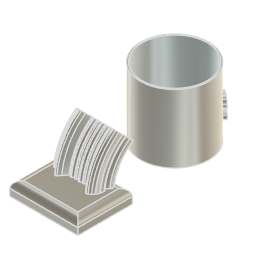
DecorativePieces (Autodesk Fusion 360 design; units mm, degrees)
Autodesk Fusion 360 part; units mm, degrees
(part 1 of 2)
sketch "Sketch1" plane through (0, 0, 0) normal (0, 0, 1) x (1, 0, 0)
  line L0 (50, 40) -> (-50, 40)
  line L1 (-50, 40) -> (-50, -40)
  line L2 (-50, -40) -> (50, -40)
  line L3 (50, -40) -> (50, 40)
  line L4 (50, 40) -> (-50, -40) construction
  line L5 (-50, 40) -> (50, -40) construction
  dimension "d1" = 100
  dimension "d2" = 80
  constraint horizontal L0
  constraint perpendicular L0 L1
  constraint parallel L0 L2
  constraint parallel L1 L3
  constraint coincident L4 origin
  constraint coincident L5 origin
  measures "d1" distance of L0.start L0.end
  measures "d2" distance of L0.end L1.end
extrude "Extrude1" add sketch "Sketch1" along normal blind 20 makes body 1
ref_plane "WorkPlane1" through (0, -40, 20) normal (0, 0.707107, 0.707107) x (1, 0, 0)
ref_plane "WorkPlane2" through (0, 30.7107, 90.7107) normal (0, 0.707107, 0.707107) x (1, 0, 0)
sketch "Sketch2" plane through (0, 60.7107, 60.7107) normal (0, 0.707107, 0.707107) x (1, 0, 0)
  line L0 (22.4639, -18.7054) -> (26.5034, -16.4275)
  spline S0 degree 2 poles (26.5034, -16.4275) (27.8398, -14.1648) (29.1838, -12.1526) knots 0 0 0 1 1 1
  spline S1 degree 2 poles (29.1838, -12.1526) (30.5277, -10.1405) (31.568, -8.8269) knots 0 0 0 1 1 1
  spline S2 degree 2 poles (31.568, -8.8269) (32.6082, -7.5133) (33.3675, -6.8223) knots 0 0 0 1 1 1
  spline S3 degree 2 poles (33.3675, -6.8223) (34.1268, -6.1314) (34.4913, -6.1314) knots 0 0 0 1 1 1
  spline S4 degree 2 poles (34.4913, -6.1314) (34.9772, -6.1314) (35.2809, -6.4579) knots 0 0 0 1 1 1
  spline S5 degree 2 poles (35.2809, -6.4579) (35.5847, -6.7844) (35.5847, -7.2248) knots 0 0 0 1 1 1
  spline S6 degree 2 poles (35.5847, -7.2248) (35.5847, -8.8648) (33.7396, -11.3326) knots 0 0 0 1 1 1
  spline S7 degree 2 poles (33.7396, -11.3326) (31.8945, -13.8003) (27.9005, -16.5793) knots 0 0 0 1 1 1
  spline S8 degree 2 poles (27.9005, -16.5793) (26.1693, -19.9051) (25.0456, -22.6234) knots 0 0 0 1 1 1
  spline S9 degree 2 poles (25.0456, -22.6234) (23.9218, -25.3417) (23.3295, -27.2703) knots 0 0 0 1 1 1
  spline S10 degree 2 poles (23.3295, -27.2703) (22.7373, -29.1989) (22.5019, -30.3683) knots 0 0 0 1 1 1
  spline S11 degree 2 poles (22.5019, -30.3683) (22.2665, -31.5376) (22.2665, -31.8565) knots 0 0 0 1 1 1
  spline S12 degree 2 poles (22.2665, -31.8565) (22.2665, -32.5095) (22.7677, -32.5095) knots 0 0 0 1 1 1
  spline S13 degree 2 poles (22.7677, -32.5095) (23.1777, -32.5095) (23.9749, -32.0387) knots 0 0 0 1 1 1
  spline S14 degree 2 poles (23.9749, -32.0387) (24.7722, -31.568) (25.6986, -30.634) knots 0 0 0 1 1 1
  spline S15 degree 2 poles (25.6986, -30.634) (26.6249, -29.7001) (27.4298, -28.47) knots 0 0 0 1 1 1
  spline S16 degree 2 poles (27.4298, -28.47) (28.2346, -27.2551) (28.8952, -25.7441) knots 0 0 0 1 1 1
  spline S17 degree 2 poles (28.8952, -25.7441) (29.5558, -24.2331) (29.9127, -22.9575) knots 0 0 0 1 1 1
  spline S18 degree 2 poles (29.9127, -22.9575) (30.2696, -21.6819) (30.2696, -20.9074) knots 0 0 0 1 1 1
  spline S19 degree 2 poles (30.2696, -20.9074) (30.2696, -20.7099) (30.2088, -20.0418) knots 0 0 0 1 1 1
  spline S20 degree 2 poles (30.2088, -20.0418) (30.0721, -20.2544) (29.8747, -20.5581) knots 0 0 0 1 1 1
  spline S21 degree 2 poles (29.8747, -20.5581) (29.6773, -20.8618) (29.3736, -21.1807) knots 0 0 0 1 1 1
  spline S22 degree 2 poles (29.3736, -21.1807) (29.0699, -21.4996) (28.7358, -21.7122) knots 0 0 0 1 1 1
  spline S23 degree 2 poles (28.7358, -21.7122) (28.5383, -21.8641) (28.265, -21.9628) knots 0 0 0 1 1 1
  spline S24 degree 2 poles (28.265, -21.9628) (27.9917, -22.0615) (27.9917, -21.94) knots 0 0 0 1 1 1
  spline S25 degree 2 poles (27.9917, -21.94) (27.9917, -21.8489) (28.8573, -20.7935) knots 0 0 0 1 1 1
  spline S26 degree 2 poles (28.8573, -20.7935) (29.7229, -19.738) (30.3607, -18.8876) knots 0 0 0 1 1 1
  spline S27 degree 2 poles (30.3607, -18.8876) (30.7251, -18.4017) (31.3326, -17.9765) knots 0 0 0 1 1 1
  spline S28 degree 2 poles (31.3326, -17.9765) (31.94, -17.5513) (32.3197, -17.5513) knots 0 0 0 1 1 1
  spline S29 degree 2 poles (32.3197, -17.5513) (32.7752, -17.5513) (32.9195, -17.9765) knots 0 0 0 1 1 1
  spline S30 degree 2 poles (32.9195, -17.9765) (33.0638, -18.4017) (33.0638, -19.328) knots 0 0 0 1 1 1
  spline S31 degree 2 poles (33.0638, -19.328) (33.0638, -21.5604) (32.2969, -24.2939) knots 0 0 0 1 1 1
  spline S32 degree 2 poles (32.2969, -24.2939) (31.53, -27.0273) (30.2392, -29.0926) knots 0 0 0 1 1 1
  spline S33 degree 2 poles (30.2392, -29.0926) (29.1913, -30.7327) (27.6727, -32.0615) knots 0 0 0 1 1 1
  spline S34 degree 2 poles (27.6727, -32.0615) (26.1541, -33.3903) (24.7191, -34.1344) knots 0 0 0 1 1 1
  spline S35 degree 2 poles (24.7191, -34.1344) (23.284, -34.8785) (22.4639, -34.8785) knots 0 0 0 1 1 1
  spline S36 degree 2 poles (22.4639, -34.8785) (21.4617, -34.8785) (20.915, -34.2483) knots 0 0 0 1 1 1
  spline S37 degree 2 poles (20.915, -34.2483) (20.3683, -33.6181) (20.3683, -32.5095) knots 0 0 0 1 1 1
  spline S38 degree 2 poles (20.3683, -32.5095) (20.3683, -31.9628) (20.4973, -31.2794) knots 0 0 0 1 1 1
  spline S39 degree 2 poles (20.4973, -31.2794) (20.6264, -30.5961) (20.8238, -29.8975) knots 0 0 0 1 1 1
  spline S40 degree 2 poles (20.8238, -29.8975) (21.0213, -29.1989) (21.5072, -27.65) knots 0 0 0 1 1 1
  spline S41 degree 2 poles (21.5072, -27.65) (21.9932, -26.101) (22.145, -25.5998) knots 0 0 0 1 1 1
  spline S42 degree 2 poles (22.145, -25.5998) (22.6158, -24.0357) (23.3827, -22.388) knots 0 0 0 1 1 1
  spline S43 degree 2 poles (23.3827, -22.388) (24.1496, -20.7403) (25.5619, -18.022) knots 0 0 0 1 1 1
  line L1 (25.5619, -18.022) -> (22.4639, -19.6925)
  line L2 (22.4639, -19.6925) -> (22.4639, -18.7054)
  line L3 (12.1724, -19.814) -> (12.1724, -18.7965)
  spline S44 degree 2 poles (12.1724, -18.7965) (13.1746, -17.8853) (13.7821, -17.5816) knots 0 0 0 1 1 1
  spline S45 degree 2 poles (13.7821, -17.5816) (14.3895, -17.2779) (15.5285, -17.3386) knots 0 0 0 1 1 1
  spline S46 degree 2 poles (15.5285, -17.3386) (17.5027, -15) (19.0061, -15) knots 0 0 0 1 1 1
  spline S47 degree 2 poles (19.0061, -15) (19.8565, -15) (20.5551, -15.5619) knots 0 0 0 1 1 1
  spline S48 degree 2 poles (20.5551, -15.5619) (21.2536, -16.1238) (21.6712, -17.0957) knots 0 0 0 1 1 1
  spline S49 degree 2 poles (21.6712, -17.0957) (22.0888, -18.0676) (22.0888, -19.2673) knots 0 0 0 1 1 1
  spline S50 degree 2 poles (22.0888, -19.2673) (22.0888, -20.2392) (21.4434, -21.4237) knots 0 0 0 1 1 1
  spline S51 degree 2 poles (21.4434, -21.4237) (20.798, -22.6082) (19.773, -23.6333) knots 0 0 0 1 1 1
  spline S52 degree 2 poles (19.773, -23.6333) (18.7479, -24.6583) (17.5786, -25.2885) knots 0 0 0 1 1 1
  spline S53 degree 2 poles (17.5786, -25.2885) (16.4093, -25.9188) (15.407, -25.9188) knots 0 0 0 1 1 1
  spline S54 degree 2 poles (15.407, -25.9188) (14.6932, -25.9188) (14.2832, -25.6986) knots 0 0 0 1 1 1
  spline S55 degree 2 poles (14.2832, -25.6986) (13.8732, -25.4784) (13.8732, -25.0835) knots 0 0 0 1 1 1
  spline S56 degree 2 poles (13.8732, -25.0835) (13.8732, -24.7798) (14.2225, -24.385) knots 0 0 0 1 1 1
  spline S57 degree 2 poles (14.2225, -24.385) (13.6454, -24.2635) (13.4328, -23.9825) knots 0 0 0 1 1 1
  spline S58 degree 2 poles (13.4328, -23.9825) (13.2202, -23.7016) (13.2202, -22.9575) knots 0 0 0 1 1 1
  spline S59 degree 2 poles (13.2202, -22.9575) (13.2202, -22.2285) (13.5619, -21.12) knots 0 0 0 1 1 1
  spline S60 degree 2 poles (13.5619, -21.12) (13.9036, -20.0114) (14.4958, -19.0395) knots 0 0 0 1 1 1
  line L4 (14.4958, -19.0395) -> (14.2225, -18.7661)
  line L5 (14.2225, -18.7661) -> (13.9947, -18.7661)
  spline S61 degree 2 poles (13.9947, -18.7661) (13.7365, -18.7661) (13.486, -18.8952) knots 0 0 0 1 1 1
  spline S62 degree 2 poles (13.486, -18.8952) (13.2354, -19.0243) (13.038, -19.1686) knots 0 0 0 1 1 1
  spline S63 degree 2 poles (13.038, -19.1686) (12.8405, -19.3128) (12.1724, -19.814) knots 0 0 0 1 1 1
  spline S64 degree 2 poles (15.3007, -23.8079) (16.5611, -23.0486) (17.4571, -22.4336) knots 0 0 0 1 1 1
  spline S65 degree 2 poles (17.4571, -22.4336) (18.3531, -21.8185) (18.9757, -21.1883) knots 0 0 0 1 1 1
  spline S66 degree 2 poles (18.9757, -21.1883) (19.5983, -20.5581) (19.8109, -19.9203) knots 0 0 0 1 1 1
  spline S67 degree 2 poles (19.8109, -19.9203) (20.1906, -18.2194) (20.1906, -18.0828) knots 0 0 0 1 1 1
  spline S68 degree 2 poles (20.1906, -18.0828) (20.1906, -17.0805) (18.7935, -17.0805) knots 0 0 0 1 1 1
  spline S69 degree 2 poles (18.7935, -17.0805) (18.1405, -17.0805) (16.6067, -18.2043) knots 0 0 0 1 1 1
  spline S70 degree 2 poles (16.6067, -18.2043) (16.8648, -18.918) (16.8648, -19.571) knots 0 0 0 1 1 1
  spline S71 degree 2 poles (16.8648, -19.571) (16.8648, -20.5277) (16.47, -21.5224) knots 0 0 0 1 1 1
  spline S72 degree 2 poles (16.47, -21.5224) (16.0752, -22.5171) (15.3007, -23.8079) knots 0 0 0 1 1 1
  spline S73 degree 2 poles (1.4708, -22.5323) (4.1435, -19.5558) (4.1435, -18.3865) knots 0 0 0 1 1 1
  spline S74 degree 2 poles (4.1435, -18.3865) (4.1435, -17.7335) (3.612, -17.7335) knots 0 0 0 1 1 1
  spline S75 degree 2 poles (3.612, -17.7335) (3.1716, -17.7335) (2.4655, -18.1967) knots 0 0 0 1 1 1
  spline S76 degree 2 poles (2.4655, -18.1967) (1.7593, -18.6598) (0.2559, -19.8443) knots 0 0 0 1 1 1
  line L6 (0.2559, -19.8443) -> (0.2559, -18.7965)
  spline S77 degree 2 poles (0.2559, -18.7965) (2.4123, -16.6705) (3.5664, -15.7289) knots 0 0 0 1 1 1
  spline S78 degree 2 poles (3.5664, -15.7289) (4.7206, -14.7874) (5.4495, -14.7874) knots 0 0 0 1 1 1
  spline S79 degree 2 poles (5.4495, -14.7874) (6.6948, -14.7874) (6.6948, -16.4275) knots 0 0 0 1 1 1
  spline S80 degree 2 poles (6.6948, -16.4275) (6.6948, -16.9134) (6.5429, -17.3842) knots 0 0 0 1 1 1
  spline S81 degree 2 poles (6.5429, -17.3842) (6.391, -17.855) (6.1253, -18.3637) knots 0 0 0 1 1 1
  spline S82 degree 2 poles (6.1253, -18.3637) (5.8595, -18.8724) (5.3128, -19.8216) knots 0 0 0 1 1 1
  spline S83 degree 2 poles (5.3128, -19.8216) (4.7661, -20.7707) (4.0524, -21.9704) knots 0 0 0 1 1 1
  spline S84 degree 2 poles (4.0524, -21.9704) (4.918, -21.53) (6.224, -20.224) knots 0 0 0 1 1 1
  spline S85 degree 2 poles (6.224, -20.224) (7.0744, -19.4039) (7.6667, -18.6674) knots 0 0 0 1 1 1
  spline S86 degree 2 poles (7.6667, -18.6674) (8.2589, -17.9309) (8.9347, -17.0273) knots 0 0 0 1 1 1
  spline S87 degree 2 poles (8.9347, -17.0273) (9.6105, -16.1238) (9.9218, -15.8125) knots 0 0 0 1 1 1
  spline S88 degree 2 poles (9.9218, -15.8125) (10.2331, -15.5011) (10.552, -15.5011) knots 0 0 0 1 1 1
  spline S89 degree 2 poles (10.552, -15.5011) (11.038, -15.5011) (11.448, -16.5186) knots 0 0 0 1 1 1
  spline S90 degree 2 poles (11.448, -16.5186) (11.858, -17.5361) (11.858, -18.8876) knots 0 0 0 1 1 1
  spline S91 degree 2 poles (11.858, -18.8876) (11.858, -19.7229) (11.6682, -20.1936) knots 0 0 0 1 1 1
  spline S92 degree 2 poles (11.6682, -20.1936) (11.4784, -20.6644) (10.9165, -21.53) knots 0 0 0 1 1 1
  spline S93 degree 2 poles (10.9165, -21.53) (9.8686, -23.1397) (9.1093, -23.8914) knots 0 0 0 1 1 1
  spline S94 degree 2 poles (9.1093, -23.8914) (8.35, -24.6431) (7.6515, -24.6431) knots 0 0 0 1 1 1
  spline S95 degree 2 poles (7.6515, -24.6431) (7.1655, -24.6431) (6.8694, -24.4761) knots 0 0 0 1 1 1
  spline S96 degree 2 poles (6.8694, -24.4761) (6.5733, -24.309) (6.5733, -23.9598) knots 0 0 0 1 1 1
  spline S97 degree 2 poles (6.5733, -23.9598) (6.5733, -23.8079) (6.6644, -23.6409) knots 0 0 0 1 1 1
  spline S98 degree 2 poles (6.6644, -23.6409) (6.7555, -23.4738) (6.8694, -23.3371) knots 0 0 0 1 1 1
  spline S99 degree 2 poles (6.8694, -23.3371) (6.9833, -23.2005) (7.3478, -22.8056) knots 0 0 0 1 1 1
  spline S100 degree 2 poles (7.3478, -22.8056) (9.7472, -20.1481) (9.7472, -19.3584) knots 0 0 0 1 1 1
  spline S101 degree 2 poles (9.7472, -19.3584) (9.7472, -18.918) (9.4586, -18.918) knots 0 0 0 1 1 1
  spline S102 degree 2 poles (9.4586, -18.918) (9.2764, -18.918) (8.7525, -19.5027) knots 0 0 0 1 1 1
  spline S103 degree 2 poles (8.7525, -19.5027) (8.2286, -20.0873) (7.4009, -21.0364) knots 0 0 0 1 1 1
  spline S104 degree 2 poles (7.4009, -21.0364) (6.5733, -21.9856) (5.4419, -23.0182) knots 0 0 0 1 1 1
  spline S105 degree 2 poles (5.4419, -23.0182) (4.3106, -24.0509) (2.8679, -25.0076) knots 0 0 0 1 1 1
  spline S106 degree 2 poles (2.8679, -25.0076) (2.063, -25.5695) (1.5315, -25.5695) knots 0 0 0 1 1 1
  spline S107 degree 2 poles (1.5315, -25.5695) (1.2885, -25.5695) (1.0532, -24.9013) knots 0 0 0 1 1 1
  spline S108 degree 2 poles (1.0532, -24.9013) (0.8178, -24.2331) (0.8178, -23.5497) knots 0 0 0 1 1 1
  spline S109 degree 2 poles (0.8178, -23.5497) (0.8178, -23.2156) (1.4708, -22.5323) knots 0 0 0 1 1 1
  spline S110 degree 2 poles (-10.385, -22.5323) (-7.7122, -19.5558) (-7.7122, -18.3865) knots 0 0 0 1 1 1
  spline S111 degree 2 poles (-7.7122, -18.3865) (-7.7122, -17.7335) (-8.2437, -17.7335) knots 0 0 0 1 1 1
  spline S112 degree 2 poles (-8.2437, -17.7335) (-8.6841, -17.7335) (-9.3903, -18.1967) knots 0 0 0 1 1 1
  spline S113 degree 2 poles (-9.3903, -18.1967) (-10.0964, -18.6598) (-11.5998, -19.8443) knots 0 0 0 1 1 1
  line L7 (-11.5998, -19.8443) -> (-11.5998, -18.7965)
  spline S114 degree 2 poles (-11.5998, -18.7965) (-9.4434, -16.6705) (-8.2893, -15.7289) knots 0 0 0 1 1 1
  spline S115 degree 2 poles (-8.2893, -15.7289) (-7.1352, -14.7874) (-6.4062, -14.7874) knots 0 0 0 1 1 1
  spline S116 degree 2 poles (-6.4062, -14.7874) (-5.161, -14.7874) (-5.161, -16.4275) knots 0 0 0 1 1 1
  spline S117 degree 2 poles (-5.161, -16.4275) (-5.161, -16.9134) (-5.3128, -17.3842) knots 0 0 0 1 1 1
  spline S118 degree 2 poles (-5.3128, -17.3842) (-5.4647, -17.855) (-5.7304, -18.3637) knots 0 0 0 1 1 1
  spline S119 degree 2 poles (-5.7304, -18.3637) (-5.9962, -18.8724) (-6.5429, -19.8216) knots 0 0 0 1 1 1
  spline S120 degree 2 poles (-6.5429, -19.8216) (-7.0896, -20.7707) (-7.8033, -21.9704) knots 0 0 0 1 1 1
  spline S121 degree 2 poles (-7.8033, -21.9704) (-6.9377, -21.53) (-5.6317, -20.224) knots 0 0 0 1 1 1
  spline S122 degree 2 poles (-5.6317, -20.224) (-4.7813, -19.4039) (-4.1891, -18.6674) knots 0 0 0 1 1 1
  spline S123 degree 2 poles (-4.1891, -18.6674) (-3.5968, -17.9309) (-2.921, -17.0273) knots 0 0 0 1 1 1
  spline S124 degree 2 poles (-2.921, -17.0273) (-2.2452, -16.1238) (-1.9339, -15.8125) knots 0 0 0 1 1 1
  spline S125 degree 2 poles (-1.9339, -15.8125) (-1.6226, -15.5011) (-1.3037, -15.5011) knots 0 0 0 1 1 1
  spline S126 degree 2 poles (-1.3037, -15.5011) (-0.8178, -15.5011) (-0.4077, -16.5186) knots 0 0 0 1 1 1
  spline S127 degree 2 poles (-0.4077, -16.5186) (0.0023, -17.5361) (0.0023, -18.8876) knots 0 0 0 1 1 1
  spline S128 degree 2 poles (0.0023, -18.8876) (0.0023, -19.7229) (-0.1875, -20.1936) knots 0 0 0 1 1 1
  spline S129 degree 2 poles (-0.1875, -20.1936) (-0.3774, -20.6644) (-0.9393, -21.53) knots 0 0 0 1 1 1
  spline S130 degree 2 poles (-0.9393, -21.53) (-1.9871, -23.1397) (-2.7464, -23.8914) knots 0 0 0 1 1 1
  spline S131 degree 2 poles (-2.7464, -23.8914) (-3.5057, -24.6431) (-4.2042, -24.6431) knots 0 0 0 1 1 1
  spline S132 degree 2 poles (-4.2042, -24.6431) (-4.6902, -24.6431) (-4.9863, -24.4761) knots 0 0 0 1 1 1
  spline S133 degree 2 poles (-4.9863, -24.4761) (-5.2825, -24.309) (-5.2825, -23.9598) knots 0 0 0 1 1 1
  spline S134 degree 2 poles (-5.2825, -23.9598) (-5.2825, -23.8079) (-5.1913, -23.6409) knots 0 0 0 1 1 1
  spline S135 degree 2 poles (-5.1913, -23.6409) (-5.1002, -23.4738) (-4.9863, -23.3371) knots 0 0 0 1 1 1
  spline S136 degree 2 poles (-4.9863, -23.3371) (-4.8724, -23.2005) (-4.508, -22.8056) knots 0 0 0 1 1 1
  spline S137 degree 2 poles (-4.508, -22.8056) (-2.1086, -20.1481) (-2.1086, -19.3584) knots 0 0 0 1 1 1
  spline S138 degree 2 poles (-2.1086, -19.3584) (-2.1086, -18.918) (-2.3971, -18.918) knots 0 0 0 1 1 1
  spline S139 degree 2 poles (-2.3971, -18.918) (-2.5793, -18.918) (-3.1033, -19.5027) knots 0 0 0 1 1 1
  spline S140 degree 2 poles (-3.1033, -19.5027) (-3.6272, -20.0873) (-4.4548, -21.0364) knots 0 0 0 1 1 1
  spline S141 degree 2 poles (-4.4548, -21.0364) (-5.2825, -21.9856) (-6.4138, -23.0182) knots 0 0 0 1 1 1
  spline S142 degree 2 poles (-6.4138, -23.0182) (-7.5452, -24.0509) (-8.9878, -25.0076) knots 0 0 0 1 1 1
  spline S143 degree 2 poles (-8.9878, -25.0076) (-9.7927, -25.5695) (-10.3242, -25.5695) knots 0 0 0 1 1 1
  spline S144 degree 2 poles (-10.3242, -25.5695) (-10.5672, -25.5695) (-10.8026, -24.9013) knots 0 0 0 1 1 1
  spline S145 degree 2 poles (-10.8026, -24.9013) (-11.038, -24.2331) (-11.038, -23.5497) knots 0 0 0 1 1 1
  spline S146 degree 2 poles (-11.038, -23.5497) (-11.038, -23.2156) (-10.385, -22.5323) knots 0 0 0 1 1 1
  line L8 (-23.3645, -19.7836) -> (-23.3645, -18.8269)
  spline S147 degree 2 poles (-23.3645, -18.8269) (-22.0433, -17.4753) (-21.079, -16.6173) knots 0 0 0 1 1 1
  spline S148 degree 2 poles (-21.079, -16.6173) (-20.1146, -15.7593) (-19.3933, -15.3189) knots 0 0 0 1 1 1
  spline S149 degree 2 poles (-19.3933, -15.3189) (-18.672, -14.8785) (-18.1708, -14.8785) knots 0 0 0 1 1 1
  spline S150 degree 2 poles (-18.1708, -14.8785) (-16.9863, -14.8785) (-16.9863, -16.2756) knots 0 0 0 1 1 1
  spline S151 degree 2 poles (-16.9863, -16.2756) (-16.9863, -17.3994) (-17.7228, -18.88) knots 0 0 0 1 1 1
  spline S152 degree 2 poles (-17.7228, -18.88) (-18.4594, -20.3607) (-19.8413, -22.3652) knots 0 0 0 1 1 1
  spline S153 degree 2 poles (-19.8413, -22.3652) (-19.1579, -21.9856) (-18.5505, -21.492) knots 0 0 0 1 1 1
  spline S154 degree 2 poles (-18.5505, -21.492) (-17.943, -20.9985) (-17.4723, -20.4594) knots 0 0 0 1 1 1
  spline S155 degree 2 poles (-17.4723, -20.4594) (-17.0015, -19.9203) (-16.6826, -19.5406) knots 0 0 0 1 1 1
  spline S156 degree 2 poles (-16.6826, -19.5406) (-15.6955, -18.432) (-14.7844, -17.2703) knots 0 0 0 1 1 1
  spline S157 degree 2 poles (-14.7844, -17.2703) (-13.8732, -16.1086) (-13.5543, -15.7593) knots 0 0 0 1 1 1
  spline S158 degree 2 poles (-13.5543, -15.7593) (-13.2354, -15.41) (-12.9468, -15.41) knots 0 0 0 1 1 1
  spline S159 degree 2 poles (-12.9468, -15.41) (-11.7623, -15.41) (-11.7623, -18.3257) knots 0 0 0 1 1 1
  spline S160 degree 2 poles (-11.7623, -18.3257) (-11.7623, -19.2825) (-12.0509, -20.4366) knots 0 0 0 1 1 1
  spline S161 degree 2 poles (-12.0509, -20.4366) (-12.3394, -21.5907) (-13.5998, -23.489) knots 0 0 0 1 1 1
  spline S162 degree 2 poles (-13.5998, -23.489) (-16.2574, -27.4677) (-18.1481, -29.9962) knots 0 0 0 1 1 1
  spline S163 degree 2 poles (-18.1481, -29.9962) (-20.0387, -32.5247) (-21.284, -33.8231) knots 0 0 0 1 1 1
  spline S164 degree 2 poles (-21.284, -33.8231) (-22.5292, -35.1215) (-22.9544, -35.0911) knots 0 0 0 1 1 1
  spline S165 degree 2 poles (-22.9544, -35.0911) (-23.4859, -35.0456) (-23.8124, -34.8785) knots 0 0 0 1 1 1
  spline S166 degree 2 poles (-23.8124, -34.8785) (-24.1389, -34.7115) (-24.1389, -34.4989) knots 0 0 0 1 1 1
  spline S167 degree 2 poles (-24.1389, -34.4989) (-24.1389, -34.1192) (-23.615, -33.246) knots 0 0 0 1 1 1
  spline S168 degree 2 poles (-23.615, -33.246) (-23.0911, -32.3728) (-21.8155, -30.5201) knots 0 0 0 1 1 1
  spline S169 degree 2 poles (-21.8155, -30.5201) (-20.4336, -28.5611) (-19.8565, -27.7639) knots 0 0 0 1 1 1
  spline S170 degree 2 poles (-19.8565, -27.7639) (-19.2794, -26.9666) (-18.1329, -25.5011) knots 0 0 0 1 1 1
  spline S171 degree 2 poles (-18.1329, -25.5011) (-16.9863, -24.0357) (-16.0372, -22.8891) knots 0 0 0 1 1 1
  spline S172 degree 2 poles (-16.0372, -22.8891) (-15.0881, -21.7426) (-13.8732, -20.4062) knots 0 0 0 1 1 1
  line L9 (-13.8732, -20.4062) -> (-13.8732, -18.5839)
  spline S173 degree 2 poles (-13.8732, -18.5839) (-15.9081, -20.8466) (-17.3963, -22.2893) knots 0 0 0 1 1 1
  spline S174 degree 2 poles (-17.3963, -22.2893) (-18.8846, -23.732) (-19.9172, -24.4685) knots 0 0 0 1 1 1
  spline S175 degree 2 poles (-19.9172, -24.4685) (-20.9499, -25.205) (-21.4358, -25.205) knots 0 0 0 1 1 1
  spline S176 degree 2 poles (-21.4358, -25.205) (-21.8914, -25.205) (-22.2863, -24.6659) knots 0 0 0 1 1 1
  spline S177 degree 2 poles (-22.2863, -24.6659) (-22.6811, -24.1268) (-22.6811, -23.7775) knots 0 0 0 1 1 1
  spline S178 degree 2 poles (-22.6811, -23.7775) (-22.6811, -23.6257) (-22.5292, -23.3979) knots 0 0 0 1 1 1
  spline S179 degree 2 poles (-22.5292, -23.3979) (-21.4358, -22.0919) (-20.7904, -21.2339) knots 0 0 0 1 1 1
  spline S180 degree 2 poles (-20.7904, -21.2339) (-20.145, -20.3759) (-19.7957, -19.7001) knots 0 0 0 1 1 1
  spline S181 degree 2 poles (-19.7957, -19.7001) (-19.4465, -19.0243) (-19.4465, -18.5383) knots 0 0 0 1 1 1
  spline S182 degree 2 poles (-19.4465, -18.5383) (-19.4465, -17.8246) (-20.1298, -17.8246) knots 0 0 0 1 1 1
  spline S183 degree 2 poles (-20.1298, -17.8246) (-20.8588, -17.8246) (-23.3645, -19.7836) knots 0 0 0 1 1 1
  line L10 (-30.8618, -19.1913) -> (-28.1587, -16.8983)
  spline S184 degree 2 poles (-28.1587, -16.8983) (-26.2301, -15.2126) (-25.5771, -15.2126) knots 0 0 0 1 1 1
  spline S185 degree 2 poles (-25.5771, -15.2126) (-24.9848, -15.2126) (-24.3318, -16.5718) knots 0 0 0 1 1 1
  spline S186 degree 2 poles (-24.3318, -16.5718) (-23.6788, -17.9309) (-23.6788, -18.9484) knots 0 0 0 1 1 1
  spline S187 degree 2 poles (-23.6788, -18.9484) (-23.6788, -19.814) (-23.9446, -20.4138) knots 0 0 0 1 1 1
  spline S188 degree 2 poles (-23.9446, -20.4138) (-24.2103, -21.0137) (-24.8633, -21.9704) knots 0 0 0 1 1 1
  spline S189 degree 2 poles (-24.8633, -21.9704) (-25.7897, -23.2612) (-26.6401, -24.1572) knots 0 0 0 1 1 1
  spline S190 degree 2 poles (-26.6401, -24.1572) (-27.4905, -25.0532) (-28.1435, -25.5467) knots 0 0 0 1 1 1
  spline S191 degree 2 poles (-28.1435, -25.5467) (-28.7965, -26.0402) (-29.0547, -26.0402) knots 0 0 0 1 1 1
  spline S192 degree 2 poles (-29.0547, -26.0402) (-29.4647, -26.0402) (-29.8519, -25.615) knots 0 0 0 1 1 1
  spline S193 degree 2 poles (-29.8519, -25.615) (-30.2392, -25.1898) (-30.2392, -24.7342) knots 0 0 0 1 1 1
  spline S194 degree 2 poles (-30.2392, -24.7342) (-30.2392, -24.4457) (-29.8216, -23.8079) knots 0 0 0 1 1 1
  spline S195 degree 2 poles (-29.8216, -23.8079) (-29.4039, -23.1701) (-28.5004, -22.1906) knots 0 0 0 1 1 1
  spline S196 degree 2 poles (-28.5004, -22.1906) (-27.5968, -21.2111) (-25.9871, -19.8443) knots 0 0 0 1 1 1
  line L11 (-25.9871, -19.8443) -> (-25.6986, -19.0091)
  spline S197 degree 2 poles (-25.6986, -19.0091) (-25.5771, -18.7661) (-25.5771, -18.5839) knots 0 0 0 1 1 1
  spline S198 degree 2 poles (-25.5771, -18.5839) (-25.5771, -18.1739) (-25.9871, -18.1739) knots 0 0 0 1 1 1
  spline S199 degree 2 poles (-25.9871, -18.1739) (-26.4123, -18.1739) (-27.984, -19.2521) knots 0 0 0 1 1 1
  spline S200 degree 2 poles (-27.984, -19.2521) (-29.5558, -20.3303) (-31.3933, -22.1526) knots 0 0 0 1 1 1
  spline S201 degree 2 poles (-31.3933, -22.1526) (-32.1071, -22.8664) (-32.5778, -23.4131) knots 0 0 0 1 1 1
  spline S202 degree 2 poles (-32.5778, -23.4131) (-33.0486, -23.9598) (-33.4282, -24.4381) knots 0 0 0 1 1 1
  spline S203 degree 2 poles (-33.4282, -24.4381) (-33.8079, -24.9165) (-34.0585, -25.1595) knots 0 0 0 1 1 1
  spline S204 degree 2 poles (-34.0585, -25.1595) (-34.309, -25.4024) (-34.5064, -25.4176) knots 0 0 0 1 1 1
  spline S205 degree 2 poles (-34.5064, -25.4176) (-34.8861, -25.4632) (-35.0987, -25.0987) knots 0 0 0 1 1 1
  spline S206 degree 2 poles (-35.0987, -25.0987) (-35.3113, -24.7342) (-35.3113, -24.0205) knots 0 0 0 1 1 1
  spline S207 degree 2 poles (-35.3113, -24.0205) (-35.3113, -23.6105) (-34.9468, -22.9954) knots 0 0 0 1 1 1
  spline S208 degree 2 poles (-34.9468, -22.9954) (-34.5824, -22.3804) (-33.5801, -20.8998) knots 0 0 0 1 1 1
  spline S209 degree 2 poles (-33.5801, -20.8998) (-32.5778, -19.4191) (-31.5831, -17.8322) knots 0 0 0 1 1 1
  spline S210 degree 2 poles (-31.5831, -17.8322) (-30.5884, -16.2453) (-29.5558, -14.2559) knots 0 0 0 1 1 1
  spline S211 degree 2 poles (-29.5558, -14.2559) (-29.6014, -14.3014) (-30.4897, -15.167) knots 0 0 0 1 1 1
  spline S212 degree 2 poles (-30.4897, -15.167) (-31.3781, -16.0327) (-32.3652, -16.9742) knots 0 0 0 1 1 1
  spline S213 degree 2 poles (-32.3652, -16.9742) (-33.3523, -17.9157) (-33.9901, -18.4852) knots 0 0 0 1 1 1
  spline S214 degree 2 poles (-33.9901, -18.4852) (-34.6279, -19.0547) (-35.5847, -19.814) knots 0 0 0 1 1 1
  line L12 (-35.5847, -19.814) -> (-35.5847, -18.7965)
  spline S215 degree 2 poles (-35.5847, -18.7965) (-33.5345, -16.5945) (-31.8717, -14.6204) knots 0 0 0 1 1 1
  spline S216 degree 2 poles (-31.8717, -14.6204) (-30.2088, -12.6462) (-29.3052, -11.4617) knots 0 0 0 1 1 1
  spline S217 degree 2 poles (-29.3052, -11.4617) (-28.4017, -10.2771) (-28.2498, -10.0797) knots 0 0 0 1 1 1
  spline S218 degree 2 poles (-28.2498, -10.0797) (-27.8398, -9.5482) (-27.5133, -9.085) knots 0 0 0 1 1 1
  spline S219 degree 2 poles (-27.5133, -9.085) (-27.1868, -8.6219) (-26.9666, -8.3713) knots 0 0 0 1 1 1
  spline S220 degree 2 poles (-26.9666, -8.3713) (-26.7464, -8.1207) (-26.6097, -8.1207) knots 0 0 0 1 1 1
  spline S221 degree 2 poles (-26.6097, -8.1207) (-26.2908, -8.1207) (-26.0402, -8.7509) knots 0 0 0 1 1 1
  spline S222 degree 2 poles (-26.0402, -8.7509) (-25.7897, -9.3812) (-25.7897, -9.8671) knots 0 0 0 1 1 1
  spline S223 degree 2 poles (-25.7897, -9.8671) (-25.7897, -10.3075) (-25.9567, -10.6416) knots 0 0 0 1 1 1
  spline S224 degree 2 poles (-25.9567, -10.6416) (-27.0501, -13.1017) (-30.8618, -19.1913) knots 0 0 0 1 1 1
sketch "Sketch3" plane through (0, 0, 0) normal (1, 0, 0) x (0, 1, 0)
  arc A0 (35.8975, 85.5238) -> (0, 0) centre (90.4071, 12.3485) ccw
  point P0 (35.8975, 85.5238)
  constraint coincident P0 A0.start
  constraint coincident A0.end origin
sweep "Sweep1" add profiles "Sketch2" path "Sketch3" along A0 section 1 bodies 1
fillet "Fillet1" radius 10 4 edges at (-50, 0, 20) (0, 40, 20) (0, -40, 20) (50, 0, 20) on bodies 1
cylinder "CylinderPrimitive1" add diameter 100 height 100 placed x (1, 0, 0) y (0, 1, 0) z (0, 0, 1) at (0, 152, 0) separate body makes body 2
ref_plane "WorkPlane3" through (0, 220, 0) normal (0, 1, 0) x (0, 0, 1)
sketch "Sketch5" plane through (0, 220, 0) normal (0, 1, 0) x (1, 0, 0)
  line L0 (22.3691, -35.3762) -> (26.3747, -33.0392)
  spline S0 degree 2 poles (26.3747, -33.0392) (27.6777, -30.7571) (28.9919, -28.7254) knots 0 0 0 1 1 1
  spline S1 degree 2 poles (28.9919, -28.7254) (30.3062, -26.6938) (31.327, -25.365) knots 0 0 0 1 1 1
  spline S2 degree 2 poles (31.327, -25.365) (32.3479, -24.0363) (33.097, -23.3343) knots 0 0 0 1 1 1
  spline S3 degree 2 poles (33.097, -23.3343) (33.846, -22.6322) (34.2105, -22.6269) knots 0 0 0 1 1 1
  spline S4 degree 2 poles (34.2105, -22.6269) (34.6964, -22.6197) (35.0048, -22.9417) knots 0 0 0 1 1 1
  spline S5 degree 2 poles (35.0048, -22.9417) (35.3133, -23.2637) (35.3198, -23.7041) knots 0 0 0 1 1 1
  spline S6 degree 2 poles (35.3198, -23.7041) (35.3439, -25.344) (33.5352, -27.8386) knots 0 0 0 1 1 1
  spline S7 degree 2 poles (33.5352, -27.8386) (31.7265, -30.3331) (27.7739, -33.1705) knots 0 0 0 1 1 1
  spline S8 degree 2 poles (27.7739, -33.1705) (26.0917, -36.5213) (25.008, -39.2558) knots 0 0 0 1 1 1
  spline S9 degree 2 poles (25.008, -39.2558) (23.9242, -41.9903) (23.3604, -43.9275) knots 0 0 0 1 1 1
  spline S10 degree 2 poles (23.3604, -43.9275) (22.7965, -45.8646) (22.5783, -47.0372) knots 0 0 0 1 1 1
  spline S11 degree 2 poles (22.5783, -47.0372) (22.3601, -48.2099) (22.3648, -48.5288) knots 0 0 0 1 1 1
  spline S12 degree 2 poles (22.3648, -48.5288) (22.3744, -49.1817) (22.8755, -49.1743) knots 0 0 0 1 1 1
  spline S13 degree 2 poles (22.8755, -49.1743) (23.2855, -49.1683) (24.0757, -48.6859) knots 0 0 0 1 1 1
  spline S14 degree 2 poles (24.0757, -48.6859) (24.866, -48.2034) (25.7785, -47.256) knots 0 0 0 1 1 1
  spline S15 degree 2 poles (25.7785, -47.256) (26.6911, -46.3086) (27.4778, -45.0668) knots 0 0 0 1 1 1
  spline S16 degree 2 poles (27.4778, -45.0668) (28.2647, -43.8402) (28.903, -42.3197) knots 0 0 0 1 1 1
  spline S17 degree 2 poles (28.903, -42.3197) (29.5414, -40.7991) (29.8795, -39.5184) knots 0 0 0 1 1 1
  spline S18 degree 2 poles (29.8795, -39.5184) (30.2176, -38.2377) (30.2062, -37.4633) knots 0 0 0 1 1 1
  spline S19 degree 2 poles (30.2062, -37.4633) (30.2033, -37.2659) (30.1327, -36.5987) knots 0 0 0 1 1 1
  spline S20 degree 2 poles (30.1327, -36.5987) (29.9992, -36.8132) (29.8063, -37.1198) knots 0 0 0 1 1 1
  spline S21 degree 2 poles (29.8063, -37.1198) (29.6133, -37.4264) (29.3143, -37.7498) knots 0 0 0 1 1 1
  spline S22 degree 2 poles (29.3143, -37.7498) (29.0153, -38.0731) (28.6844, -38.2906) knots 0 0 0 1 1 1
  spline S23 degree 2 poles (28.6844, -38.2906) (28.4892, -38.4453) (28.2173, -38.548) knots 0 0 0 1 1 1
  spline S24 degree 2 poles (28.2173, -38.548) (27.9455, -38.6507) (27.9437, -38.5293) knots 0 0 0 1 1 1
  spline S25 degree 2 poles (27.9437, -38.5293) (27.9424, -38.4382) (28.7924, -37.3701) knots 0 0 0 1 1 1
  spline S26 degree 2 poles (28.7924, -37.3701) (29.6424, -36.3021) (30.2676, -35.4424) knots 0 0 0 1 1 1
  spline S27 degree 2 poles (30.2676, -35.4424) (30.6249, -34.9512) (31.2261, -34.5171) knots 0 0 0 1 1 1
  spline S28 degree 2 poles (31.2261, -34.5171) (31.8272, -34.083) (32.2068, -34.0774) knots 0 0 0 1 1 1
  spline S29 degree 2 poles (32.2068, -34.0774) (32.6623, -34.0707) (32.8128, -34.4938) knots 0 0 0 1 1 1
  spline S30 degree 2 poles (32.8128, -34.4938) (32.9633, -34.9168) (32.9769, -35.8431) knots 0 0 0 1 1 1
  spline S31 degree 2 poles (32.9769, -35.8431) (33.0097, -38.0752) (32.283, -40.8196) knots 0 0 0 1 1 1
  spline S32 degree 2 poles (32.283, -40.8196) (31.5564, -43.5641) (30.296, -45.6481) knots 0 0 0 1 1 1
  spline S33 degree 2 poles (30.296, -45.6481) (29.2724, -47.3034) (27.7735, -48.6543) knots 0 0 0 1 1 1
  spline S34 degree 2 poles (27.7735, -48.6543) (26.2745, -50.0053) (24.8505, -50.7704) knots 0 0 0 1 1 1
  spline S35 degree 2 poles (24.8505, -50.7704) (23.4265, -51.5355) (22.6066, -51.5475) knots 0 0 0 1 1 1
  spline S36 degree 2 poles (22.6066, -51.5475) (21.6044, -51.5623) (21.0485, -50.9401) knots 0 0 0 1 1 1
  spline S37 degree 2 poles (21.0485, -50.9401) (20.4926, -50.318) (20.4763, -49.2096) knots 0 0 0 1 1 1
  spline S38 degree 2 poles (20.4763, -49.2096) (20.4683, -48.6629) (20.5874, -47.9777) knots 0 0 0 1 1 1
  spline S39 degree 2 poles (20.5874, -47.9777) (20.7064, -47.2925) (20.8935, -46.5912) knots 0 0 0 1 1 1
  spline S40 degree 2 poles (20.8935, -46.5912) (21.0807, -45.8898) (21.5438, -44.3338) knots 0 0 0 1 1 1
  spline S41 degree 2 poles (21.5438, -44.3338) (22.007, -42.7779) (22.1515, -42.2746) knots 0 0 0 1 1 1
  spline S42 degree 2 poles (22.1515, -42.2746) (22.5992, -40.7037) (23.3418, -39.0449) knots 0 0 0 1 1 1
  spline S43 degree 2 poles (23.3418, -39.0449) (24.0844, -37.3861) (25.4567, -34.6474) knots 0 0 0 1 1 1
  line L1 (25.4567, -34.6474) -> (22.3836, -36.3632)
  line L2 (22.3836, -36.3632) -> (22.3691, -35.3762)
  line L3 (12.0949, -36.6358) -> (12.0799, -35.6184)
  spline S44 degree 2 poles (12.0799, -35.6184) (13.0687, -34.6926) (13.6717, -34.38) knots 0 0 0 1 1 1
  spline S45 degree 2 poles (13.6717, -34.38) (14.2746, -34.0674) (15.4143, -34.1114) knots 0 0 0 1 1 1
  spline S46 degree 2 poles (15.4143, -34.1114) (17.3539, -31.744) (18.8572, -31.722) knots 0 0 0 1 1 1
  spline S47 degree 2 poles (18.8572, -31.722) (19.7075, -31.7095) (20.4142, -32.261) knots 0 0 0 1 1 1
  spline S48 degree 2 poles (20.4142, -32.261) (21.121, -32.8126) (21.5528, -33.7783) knots 0 0 0 1 1 1
  spline S49 degree 2 poles (21.5528, -33.7783) (21.9847, -34.7439) (22.0023, -35.9435) knots 0 0 0 1 1 1
  spline S50 degree 2 poles (22.0023, -35.9435) (22.0165, -36.9153) (21.3886, -38.1092) knots 0 0 0 1 1 1
  spline S51 degree 2 poles (21.3886, -38.1092) (20.7607, -39.303) (19.7508, -40.343) knots 0 0 0 1 1 1
  spline S52 degree 2 poles (19.7508, -40.343) (18.7409, -41.383) (17.5809, -42.0303) knots 0 0 0 1 1 1
  spline S53 degree 2 poles (17.5809, -42.0303) (16.421, -42.6777) (15.4188, -42.6924) knots 0 0 0 1 1 1
  spline S54 degree 2 poles (15.4188, -42.6924) (14.7052, -42.7029) (14.2919, -42.4887) knots 0 0 0 1 1 1
  spline S55 degree 2 poles (14.2919, -42.4887) (13.8787, -42.2746) (13.8729, -41.8798) knots 0 0 0 1 1 1
  spline S56 degree 2 poles (13.8729, -41.8798) (13.8685, -41.5761) (14.2119, -41.1762) knots 0 0 0 1 1 1
  spline S57 degree 2 poles (14.2119, -41.1762) (13.6331, -41.0632) (13.4164, -40.7854) knots 0 0 0 1 1 1
  spline S58 degree 2 poles (13.4164, -40.7854) (13.1997, -40.5076) (13.1888, -39.7635) knots 0 0 0 1 1 1
  spline S59 degree 2 poles (13.1888, -39.7635) (13.1781, -39.0347) (13.5034, -37.9212) knots 0 0 0 1 1 1
  spline S60 degree 2 poles (13.5034, -37.9212) (13.8288, -36.8077) (14.4067, -35.8272) knots 0 0 0 1 1 1
  line L4 (14.4067, -35.8272) -> (14.1294, -35.5579)
  line L5 (14.1294, -35.5579) -> (13.9016, -35.5613)
  spline S61 degree 2 poles (13.9016, -35.5613) (13.6435, -35.5651) (13.3948, -35.6978) knots 0 0 0 1 1 1
  spline S62 degree 2 poles (13.3948, -35.6978) (13.1462, -35.8306) (12.9509, -35.9777) knots 0 0 0 1 1 1
  spline S63 degree 2 poles (12.9509, -35.9777) (12.7556, -36.1249) (12.0949, -36.6358) knots 0 0 0 1 1 1
  spline S64 degree 2 poles (15.2815, -40.5833) (16.5307, -39.8056) (17.4175, -39.1775) knots 0 0 0 1 1 1
  spline S65 degree 2 poles (17.4175, -39.1775) (18.3044, -38.5493) (18.9177, -37.91) knots 0 0 0 1 1 1
  spline S66 degree 2 poles (18.9177, -37.91) (19.531, -37.2707) (19.7342, -36.6299) knots 0 0 0 1 1 1
  spline S67 degree 2 poles (19.7342, -36.6299) (20.0888, -34.9237) (20.0868, -34.787) knots 0 0 0 1 1 1
  spline S68 degree 2 poles (20.0868, -34.787) (20.0721, -33.7848) (18.6751, -33.8053) knots 0 0 0 1 1 1
  spline S69 degree 2 poles (18.6751, -33.8053) (18.0222, -33.8149) (16.5051, -34.9611) knots 0 0 0 1 1 1
  spline S70 degree 2 poles (16.5051, -34.9611) (16.7737, -35.671) (16.7833, -36.3239) knots 0 0 0 1 1 1
  spline S71 degree 2 poles (16.7833, -36.3239) (16.7973, -37.2805) (16.4172, -38.2809) knots 0 0 0 1 1 1
  spline S72 degree 2 poles (16.4172, -38.2809) (16.037, -39.2813) (15.2815, -40.5833) knots 0 0 0 1 1 1
  spline S73 degree 2 poles (1.4344, -39.5109) (4.0631, -36.4955) (4.0459, -35.3263) knots 0 0 0 1 1 1
  spline S74 degree 2 poles (4.0459, -35.3263) (4.0364, -34.6734) (3.5049, -34.6812) knots 0 0 0 1 1 1
  spline S75 degree 2 poles (3.5049, -34.6812) (3.0646, -34.6877) (2.3653, -35.1612) knots 0 0 0 1 1 1
  spline S76 degree 2 poles (2.3653, -35.1612) (1.666, -35.6347) (0.1801, -36.8411) knots 0 0 0 1 1 1
  line L6 (0.1801, -36.8411) -> (0.1648, -35.7934)
  spline S77 degree 2 poles (0.1648, -35.7934) (2.2897, -33.6359) (3.4299, -32.6776) knots 0 0 0 1 1 1
  spline S78 degree 2 poles (3.4299, -32.6776) (4.5701, -31.7192) (5.2989, -31.7085) knots 0 0 0 1 1 1
  spline S79 degree 2 poles (5.2989, -31.7085) (6.5441, -31.6902) (6.5681, -33.3301) knots 0 0 0 1 1 1
  spline S80 degree 2 poles (6.5681, -33.3301) (6.5753, -33.816) (6.4304, -34.2889) knots 0 0 0 1 1 1
  spline S81 degree 2 poles (6.4304, -34.2889) (6.2854, -34.7619) (6.0272, -35.2745) knots 0 0 0 1 1 1
  spline S82 degree 2 poles (6.0272, -35.2745) (5.7689, -35.787) (5.2362, -36.7441) knots 0 0 0 1 1 1
  spline S83 degree 2 poles (5.2362, -36.7441) (4.7035, -37.7012) (4.0075, -38.9112) knots 0 0 0 1 1 1
  spline S84 degree 2 poles (4.0075, -38.9112) (4.8665, -38.4581) (6.1532, -37.1331) knots 0 0 0 1 1 1
  spline S85 degree 2 poles (6.1532, -37.1331) (6.9915, -36.3007) (7.5728, -35.5555) knots 0 0 0 1 1 1
  spline S86 degree 2 poles (7.5728, -35.5555) (8.1542, -34.8104) (8.8167, -33.897) knots 0 0 0 1 1 1
  spline S87 degree 2 poles (8.8167, -33.897) (9.4791, -32.9836) (9.7858, -32.6677) knots 0 0 0 1 1 1
  spline S88 degree 2 poles (9.7858, -32.6677) (10.0925, -32.3519) (10.4114, -32.3472) knots 0 0 0 1 1 1
  spline S89 degree 2 poles (10.4114, -32.3472) (10.8973, -32.3401) (11.3222, -33.3514) knots 0 0 0 1 1 1
  spline S90 degree 2 poles (11.3222, -33.3514) (11.7471, -34.3627) (11.767, -35.7141) knots 0 0 0 1 1 1
  spline S91 degree 2 poles (11.767, -35.7141) (11.7792, -36.5493) (11.5963, -37.0228) knots 0 0 0 1 1 1
  spline S92 degree 2 poles (11.5963, -37.0228) (11.4135, -37.4963) (10.8643, -38.37) knots 0 0 0 1 1 1
  spline S93 degree 2 poles (10.8643, -38.37) (9.8403, -39.995) (9.0921, -40.7578) knots 0 0 0 1 1 1
  spline S94 degree 2 poles (9.0921, -40.7578) (8.3439, -41.5205) (7.6454, -41.5308) knots 0 0 0 1 1 1
  spline S95 degree 2 poles (7.6454, -41.5308) (7.1595, -41.5379) (6.861, -41.3753) knots 0 0 0 1 1 1
  spline S96 degree 2 poles (6.861, -41.3753) (6.5624, -41.2126) (6.5573, -40.8633) knots 0 0 0 1 1 1
  spline S97 degree 2 poles (6.5573, -40.8633) (6.5551, -40.7115) (6.6437, -40.5431) knots 0 0 0 1 1 1
  spline S98 degree 2 poles (6.6437, -40.5431) (6.7324, -40.3748) (6.8442, -40.2364) knots 0 0 0 1 1 1
  spline S99 degree 2 poles (6.8442, -40.2364) (6.9561, -40.0981) (7.3147, -39.6979) knots 0 0 0 1 1 1
  spline S100 degree 2 poles (7.3147, -39.6979) (9.6749, -37.0054) (9.6633, -36.2159) knots 0 0 0 1 1 1
  spline S101 degree 2 poles (9.6633, -36.2159) (9.6568, -35.7755) (9.3683, -35.7797) knots 0 0 0 1 1 1
  spline S102 degree 2 poles (9.3683, -35.7797) (9.1861, -35.7824) (8.6708, -36.3747) knots 0 0 0 1 1 1
  spline S103 degree 2 poles (8.6708, -36.3747) (8.1555, -36.967) (7.3419, -37.9282) knots 0 0 0 1 1 1
  spline S104 degree 2 poles (7.3419, -37.9282) (6.5283, -38.8894) (5.4122, -39.9385) knots 0 0 0 1 1 1
  spline S105 degree 2 poles (5.4122, -39.9385) (4.2962, -40.9877) (2.8677, -41.9655) knots 0 0 0 1 1 1
  spline S106 degree 2 poles (2.8677, -41.9655) (2.0712, -42.5391) (1.5397, -42.5469) knots 0 0 0 1 1 1
  spline S107 degree 2 poles (1.5397, -42.5469) (1.2968, -42.5505) (1.0516, -41.8858) knots 0 0 0 1 1 1
  spline S108 degree 2 poles (1.0516, -41.8858) (0.8064, -41.2212) (0.7964, -40.5379) knots 0 0 0 1 1 1
  spline S109 degree 2 poles (0.7964, -40.5379) (0.7915, -40.2038) (1.4344, -39.5109) knots 0 0 0 1 1 1
  spline S110 degree 2 poles (-10.4201, -39.685) (-7.7913, -36.6697) (-7.8085, -35.5005) knots 0 0 0 1 1 1
  spline S111 degree 2 poles (-7.8085, -35.5005) (-7.8181, -34.8475) (-8.3496, -34.8553) knots 0 0 0 1 1 1
  spline S112 degree 2 poles (-8.3496, -34.8553) (-8.7899, -34.8618) (-9.4892, -35.3353) knots 0 0 0 1 1 1
  spline S113 degree 2 poles (-9.4892, -35.3353) (-10.1884, -35.8088) (-11.6743, -37.0153) knots 0 0 0 1 1 1
  line L7 (-11.6743, -37.0153) -> (-11.6897, -35.9675)
  spline S114 degree 2 poles (-11.6897, -35.9675) (-9.5647, -33.81) (-8.4245, -32.8517) knots 0 0 0 1 1 1
  spline S115 degree 2 poles (-8.4245, -32.8517) (-7.2844, -31.8933) (-6.5555, -31.8826) knots 0 0 0 1 1 1
  spline S116 degree 2 poles (-6.5555, -31.8826) (-5.3104, -31.8643) (-5.2863, -33.5042) knots 0 0 0 1 1 1
  spline S117 degree 2 poles (-5.2863, -33.5042) (-5.2792, -33.9901) (-5.4241, -34.4631) knots 0 0 0 1 1 1
  spline S118 degree 2 poles (-5.4241, -34.4631) (-5.569, -34.936) (-5.8273, -35.4486) knots 0 0 0 1 1 1
  spline S119 degree 2 poles (-5.8273, -35.4486) (-6.0855, -35.9612) (-6.6182, -36.9182) knots 0 0 0 1 1 1
  spline S120 degree 2 poles (-6.6182, -36.9182) (-7.1509, -37.8753) (-7.847, -39.0853) knots 0 0 0 1 1 1
  spline S121 degree 2 poles (-7.847, -39.0853) (-6.9879, -38.6323) (-5.7013, -37.3072) knots 0 0 0 1 1 1
  spline S122 degree 2 poles (-5.7013, -37.3072) (-4.863, -36.4748) (-4.2816, -35.7296) knots 0 0 0 1 1 1
  spline S123 degree 2 poles (-4.2816, -35.7296) (-3.7002, -34.9845) (-3.0378, -34.0711) knots 0 0 0 1 1 1
  spline S124 degree 2 poles (-3.0378, -34.0711) (-2.3754, -33.1577) (-2.0687, -32.8418) knots 0 0 0 1 1 1
  spline S125 degree 2 poles (-2.0687, -32.8418) (-1.7619, -32.526) (-1.4431, -32.5213) knots 0 0 0 1 1 1
  spline S126 degree 2 poles (-1.4431, -32.5213) (-0.9572, -32.5142) (-0.5323, -33.5255) knots 0 0 0 1 1 1
  spline S127 degree 2 poles (-0.5323, -33.5255) (-0.1073, -34.5368) (-0.0875, -35.8882) knots 0 0 0 1 1 1
  spline S128 degree 2 poles (-0.0875, -35.8882) (-0.0752, -36.7234) (-0.2581, -37.1969) knots 0 0 0 1 1 1
  spline S129 degree 2 poles (-0.2581, -37.1969) (-0.441, -37.6704) (-0.9901, -38.5442) knots 0 0 0 1 1 1
  spline S130 degree 2 poles (-0.9901, -38.5442) (-2.0142, -40.1691) (-2.7624, -40.9319) knots 0 0 0 1 1 1
  spline S131 degree 2 poles (-2.7624, -40.9319) (-3.5106, -41.6947) (-4.209, -41.7049) knots 0 0 0 1 1 1
  spline S132 degree 2 poles (-4.209, -41.7049) (-4.6949, -41.712) (-4.9935, -41.5494) knots 0 0 0 1 1 1
  spline S133 degree 2 poles (-4.9935, -41.5494) (-5.292, -41.3867) (-5.2972, -41.0374) knots 0 0 0 1 1 1
  spline S134 degree 2 poles (-5.2972, -41.0374) (-5.2994, -40.8856) (-5.2107, -40.7172) knots 0 0 0 1 1 1
  spline S135 degree 2 poles (-5.2107, -40.7172) (-5.1221, -40.5489) (-5.0102, -40.4105) knots 0 0 0 1 1 1
  spline S136 degree 2 poles (-5.0102, -40.4105) (-4.8983, -40.2722) (-4.5397, -39.8721) knots 0 0 0 1 1 1
  spline S137 degree 2 poles (-4.5397, -39.8721) (-2.1796, -37.1796) (-2.1912, -36.39) knots 0 0 0 1 1 1
  spline S138 degree 2 poles (-2.1912, -36.39) (-2.1977, -35.9496) (-2.4862, -35.9539) knots 0 0 0 1 1 1
  spline S139 degree 2 poles (-2.4862, -35.9539) (-2.6684, -35.9565) (-3.1837, -36.5488) knots 0 0 0 1 1 1
  spline S140 degree 2 poles (-3.1837, -36.5488) (-3.6989, -37.1411) (-4.5125, -38.1023) knots 0 0 0 1 1 1
  spline S141 degree 2 poles (-4.5125, -38.1023) (-5.3262, -39.0635) (-6.4422, -40.1126) knots 0 0 0 1 1 1
  spline S142 degree 2 poles (-6.4422, -40.1126) (-7.5583, -41.1618) (-8.9868, -42.1396) knots 0 0 0 1 1 1
  spline S143 degree 2 poles (-8.9868, -42.1396) (-9.7833, -42.7132) (-10.3147, -42.721) knots 0 0 0 1 1 1
  spline S144 degree 2 poles (-10.3147, -42.721) (-10.5577, -42.7246) (-10.8029, -42.0599) knots 0 0 0 1 1 1
  spline S145 degree 2 poles (-10.8029, -42.0599) (-11.048, -41.3953) (-11.0581, -40.712) knots 0 0 0 1 1 1
  spline S146 degree 2 poles (-11.0581, -40.712) (-11.063, -40.3779) (-10.4201, -39.685) knots 0 0 0 1 1 1
  line L8 (-23.4385, -37.1273) -> (-23.4526, -36.1707)
  spline S147 degree 2 poles (-23.4526, -36.1707) (-22.1514, -34.7999) (-21.1998, -33.9278) knots 0 0 0 1 1 1
  spline S148 degree 2 poles (-21.1998, -33.9278) (-20.2482, -33.0557) (-19.5334, -32.6048) knots 0 0 0 1 1 1
  spline S149 degree 2 poles (-19.5334, -32.6048) (-18.8186, -32.1538) (-18.3175, -32.1465) knots 0 0 0 1 1 1
  spline S150 degree 2 poles (-18.3175, -32.1465) (-17.1331, -32.1291) (-17.1126, -33.526) knots 0 0 0 1 1 1
  spline S151 degree 2 poles (-17.1126, -33.526) (-17.0961, -34.6497) (-17.8108, -36.141) knots 0 0 0 1 1 1
  spline S152 degree 2 poles (-17.8108, -36.141) (-18.5255, -37.6323) (-19.8779, -39.6569) knots 0 0 0 1 1 1
  spline S153 degree 2 poles (-19.8779, -39.6569) (-19.2001, -39.2672) (-18.6, -38.7648) knots 0 0 0 1 1 1
  spline S154 degree 2 poles (-18.6, -38.7648) (-17.9999, -38.2624) (-17.5371, -37.7165) knots 0 0 0 1 1 1
  spline S155 degree 2 poles (-17.5371, -37.7165) (-17.0743, -37.1705) (-16.761, -36.7862) knots 0 0 0 1 1 1
  spline S156 degree 2 poles (-16.761, -36.7862) (-15.7903, -35.6633) (-14.8963, -34.4883) knots 0 0 0 1 1 1
  spline S157 degree 2 poles (-14.8963, -34.4883) (-14.0023, -33.3133) (-13.6885, -32.9594) knots 0 0 0 1 1 1
  spline S158 degree 2 poles (-13.6885, -32.9594) (-13.3748, -32.6054) (-13.0863, -32.6012) knots 0 0 0 1 1 1
  spline S159 degree 2 poles (-13.0863, -32.6012) (-11.9019, -32.5838) (-11.8591, -35.4992) knots 0 0 0 1 1 1
  spline S160 degree 2 poles (-11.8591, -35.4992) (-11.845, -36.4558) (-12.1166, -37.6141) knots 0 0 0 1 1 1
  spline S161 degree 2 poles (-12.1166, -37.6141) (-12.3881, -38.7723) (-13.6206, -40.6889) knots 0 0 0 1 1 1
  spline S162 degree 2 poles (-13.6206, -40.6889) (-16.2194, -44.7062) (-18.0727, -47.2622) knots 0 0 0 1 1 1
  spline S163 degree 2 poles (-18.0727, -47.2622) (-19.9261, -49.8181) (-21.1521, -51.1347) knots 0 0 0 1 1 1
  spline S164 degree 2 poles (-21.1521, -51.1347) (-22.3782, -52.4513) (-22.8038, -52.4271) knots 0 0 0 1 1 1
  spline S165 degree 2 poles (-22.8038, -52.4271) (-23.3359, -52.3894) (-23.6648, -52.2271) knots 0 0 0 1 1 1
  spline S166 degree 2 poles (-23.6648, -52.2271) (-23.9937, -52.0649) (-23.9968, -51.8523) knots 0 0 0 1 1 1
  spline S167 degree 2 poles (-23.9968, -51.8523) (-24.0024, -51.4727) (-23.4914, -50.5919) knots 0 0 0 1 1 1
  spline S168 degree 2 poles (-23.4914, -50.5919) (-22.9803, -49.7111) (-21.7321, -47.8399) knots 0 0 0 1 1 1
  spline S169 degree 2 poles (-21.7321, -47.8399) (-20.3791, -45.8608) (-19.8138, -45.0552) knots 0 0 0 1 1 1
  spline S170 degree 2 poles (-19.8138, -45.0552) (-19.2485, -44.2495) (-18.1236, -42.7674) knots 0 0 0 1 1 1
  spline S171 degree 2 poles (-18.1236, -42.7674) (-16.9987, -41.2852) (-16.0665, -40.1249) knots 0 0 0 1 1 1
  spline S172 degree 2 poles (-16.0665, -40.1249) (-15.1343, -38.9645) (-13.9392, -37.6105) knots 0 0 0 1 1 1
  line L9 (-13.9392, -37.6105) -> (-13.9659, -35.7883)
  spline S173 degree 2 poles (-13.9659, -35.7883) (-15.9674, -38.0807) (-17.4343, -39.5451) knots 0 0 0 1 1 1
  spline S174 degree 2 poles (-17.4343, -39.5451) (-18.9012, -41.0094) (-19.9229, -41.761) knots 0 0 0 1 1 1
  spline S175 degree 2 poles (-19.9229, -41.761) (-20.9446, -42.5127) (-21.4305, -42.5198) knots 0 0 0 1 1 1
  spline S176 degree 2 poles (-21.4305, -42.5198) (-21.886, -42.5265) (-22.2888, -41.9932) knots 0 0 0 1 1 1
  spline S177 degree 2 poles (-22.2888, -41.9932) (-22.6915, -41.46) (-22.6966, -41.1107) knots 0 0 0 1 1 1
  spline S178 degree 2 poles (-22.6966, -41.1107) (-22.6988, -40.9589) (-22.5503, -40.7289) knots 0 0 0 1 1 1
  spline S179 degree 2 poles (-22.5503, -40.7289) (-21.4762, -39.407) (-20.8435, -38.5396) knots 0 0 0 1 1 1
  spline S180 degree 2 poles (-20.8435, -38.5396) (-20.2108, -37.6722) (-19.8714, -36.9914) knots 0 0 0 1 1 1
  spline S181 degree 2 poles (-19.8714, -36.9914) (-19.5321, -36.3105) (-19.5393, -35.8246) knots 0 0 0 1 1 1
  spline S182 degree 2 poles (-19.5393, -35.8246) (-19.5497, -35.111) (-20.233, -35.121) knots 0 0 0 1 1 1
  spline S183 degree 2 poles (-20.233, -35.121) (-20.9619, -35.1317) (-23.4385, -37.1273) knots 0 0 0 1 1 1
  line L10 (-30.9438, -36.6452) -> (-28.2746, -34.3127)
  spline S184 degree 2 poles (-28.2746, -34.3127) (-26.371, -32.5989) (-25.718, -32.5893) knots 0 0 0 1 1 1
  spline S185 degree 2 poles (-25.718, -32.5893) (-25.1258, -32.5806) (-24.453, -33.93) knots 0 0 0 1 1 1
  spline S186 degree 2 poles (-24.453, -33.93) (-23.7801, -35.2794) (-23.7651, -36.2968) knots 0 0 0 1 1 1
  spline S187 degree 2 poles (-23.7651, -36.2968) (-23.7524, -37.1623) (-24.0093, -37.766) knots 0 0 0 1 1 1
  spline S188 degree 2 poles (-24.0093, -37.766) (-24.2662, -38.3696) (-24.9051, -39.3358) knots 0 0 0 1 1 1
  spline S189 degree 2 poles (-24.9051, -39.3358) (-25.8124, -40.6401) (-26.6496, -41.5485) knots 0 0 0 1 1 1
  spline S190 degree 2 poles (-26.6496, -41.5485) (-27.4868, -42.4569) (-28.1324, -42.9599) knots 0 0 0 1 1 1
  spline S191 degree 2 poles (-28.1324, -42.9599) (-28.7781, -43.463) (-29.0362, -43.4668) knots 0 0 0 1 1 1
  spline S192 degree 2 poles (-29.0362, -43.4668) (-29.4462, -43.4728) (-29.8397, -43.0534) knots 0 0 0 1 1 1
  spline S193 degree 2 poles (-29.8397, -43.0534) (-30.2331, -42.6339) (-30.2398, -42.1784) knots 0 0 0 1 1 1
  spline S194 degree 2 poles (-30.2398, -42.1784) (-30.244, -41.8899) (-29.8358, -41.246) knots 0 0 0 1 1 1
  spline S195 degree 2 poles (-29.8358, -41.246) (-29.4276, -40.6021) (-28.5386, -39.6094) knots 0 0 0 1 1 1
  spline S196 degree 2 poles (-28.5386, -39.6094) (-27.6495, -38.6168) (-26.06, -37.2265) knots 0 0 0 1 1 1
  line L11 (-26.06, -37.2265) -> (-25.7838, -36.3872)
  spline S197 degree 2 poles (-25.7838, -36.3872) (-25.6659, -36.1424) (-25.6685, -35.9602) knots 0 0 0 1 1 1
  spline S198 degree 2 poles (-25.6685, -35.9602) (-25.6746, -35.5502) (-26.0845, -35.5563) knots 0 0 0 1 1 1
  spline S199 degree 2 poles (-26.0845, -35.5563) (-26.5097, -35.5625) (-28.0654, -36.6637) knots 0 0 0 1 1 1
  spline S200 degree 2 poles (-28.0654, -36.6637) (-29.6212, -37.7648) (-31.4317, -39.614) knots 0 0 0 1 1 1
  spline S201 degree 2 poles (-31.4317, -39.614) (-32.1349, -40.3381) (-32.5976, -40.8917) knots 0 0 0 1 1 1
  spline S202 degree 2 poles (-32.5976, -40.8917) (-33.0603, -41.4452) (-33.4329, -41.9291) knots 0 0 0 1 1 1
  spline S203 degree 2 poles (-33.4329, -41.9291) (-33.8055, -42.413) (-34.0524, -42.6596) knots 0 0 0 1 1 1
  spline S204 degree 2 poles (-34.0524, -42.6596) (-34.2994, -42.9062) (-34.4966, -42.9243) knots 0 0 0 1 1 1
  spline S205 degree 2 poles (-34.4966, -42.9243) (-34.8755, -42.9755) (-35.0935, -42.6142) knots 0 0 0 1 1 1
  spline S206 degree 2 poles (-35.0935, -42.6142) (-35.3114, -42.2528) (-35.3219, -41.5392) knots 0 0 0 1 1 1
  spline S207 degree 2 poles (-35.3219, -41.5392) (-35.3279, -41.1292) (-34.9725, -40.5089) knots 0 0 0 1 1 1
  spline S208 degree 2 poles (-34.9725, -40.5089) (-34.6171, -39.8886) (-33.6367, -38.3934) knots 0 0 0 1 1 1
  spline S209 degree 2 poles (-33.6367, -38.3934) (-32.6563, -36.8982) (-31.685, -35.2968) knots 0 0 0 1 1 1
  spline S210 degree 2 poles (-31.685, -35.2968) (-30.7137, -33.6954) (-29.7104, -31.6911) knots 0 0 0 1 1 1
  spline S211 degree 2 poles (-29.7104, -31.6911) (-29.7553, -31.7373) (-30.6309, -32.6159) knots 0 0 0 1 1 1
  spline S212 degree 2 poles (-30.6309, -32.6159) (-31.5064, -33.4944) (-32.4796, -34.4504) knots 0 0 0 1 1 1
  spline S213 degree 2 poles (-32.4796, -34.4504) (-33.4527, -35.4063) (-34.0821, -35.9851) knots 0 0 0 1 1 1
  spline S214 degree 2 poles (-34.0821, -35.9851) (-34.7115, -36.5638) (-35.657, -37.3371) knots 0 0 0 1 1 1